Autodesk Fusion 360 part; units mm, degrees
(part 5 of 7)
  spline S1268 degree 3 poles (-26.8573, 27.0141) (-26.7843, 26.9991) (-26.7112, 26.9819) (-26.6403, 26.9626) knots 0 0 0 0 1 1 1 1
  spline S1269 degree 3 poles (-26.6403, 26.9626) (-26.7779, 27.1452) (-27.2419, 27.8115) (-27.359, 27.934) knots 0 0 0 0 1 1 1 1
  spline S1270 degree 3 poles (-27.359, 27.934) (-27.4804, 28.0619) (-27.4042, 28.1242) (-27.2967, 28.0114) knots 0 0 0 0 1 1 1 1
  spline S1271 degree 3 poles (-27.2967, 28.0114) (-27.2076, 27.9179) (-26.506, 27.1528) (-26.2332, 26.8132) knots 0 0 0 0 1 1 1 1
  spline S1272 degree 3 poles (-26.2332, 26.8132) (-26.159, 26.7767) (-26.086, 26.738) (-26.0172, 26.6939) knots 0 0 0 0 1 1 1 1
  line L670 (-26.0172, 26.6939) -> (-25.9807, 26.6692)
  spline S1273 degree 3 poles (-25.9807, 26.6692) (-26.0989, 26.8454) (-26.6231, 27.488) (-26.7305, 27.6535) knots 0 0 0 0 1 1 1 1
  spline S1274 degree 3 poles (-26.7305, 27.6535) (-26.8477, 27.833) (-26.7757, 27.8384) (-26.7037, 27.7492) knots 0 0 0 0 1 1 1 1
  spline S1275 degree 3 poles (-26.7037, 27.7492) (-26.6317, 27.661) (-25.8883, 26.8583) (-25.7755, 26.7412) knots 0 0 0 0 1 1 1 1
  spline S1276 degree 3 poles (-25.7755, 26.7412) (-25.7562, 26.7734) (-25.7368, 26.8089) (-25.7174, 26.8487) knots 0 0 0 0 1 1 1 1
  spline S1277 degree 3 poles (-25.7174, 26.8487) (-25.8603, 27.0163) (-26.5586, 27.8749) (-26.6532, 28.006) knots 0 0 0 0 1 1 1 1
  spline S1278 degree 3 poles (-26.6532, 28.006) (-26.7541, 28.1446) (-26.635, 28.1511) (-26.5802, 28.0672) knots 0 0 0 0 1 1 1 1
  spline S1279 degree 3 poles (-26.5802, 28.0672) (-26.5286, 27.9888) (-25.8356, 27.1882) (-25.6584, 26.9894) knots 0 0 0 0 1 1 1 1
  spline S1280 degree 3 poles (-25.6584, 26.9894) (-25.6391, 27.0335) (-25.6241, 27.0808) (-25.6058, 27.1324) knots 0 0 0 0 1 1 1 1
  spline S1281 degree 3 poles (-25.6058, 27.1324) (-25.6895, 27.2334) (-26.202, 27.8953) (-26.2793, 27.9888) knots 0 0 0 0 1 1 1 1
  spline S1282 degree 3 poles (-26.2793, 27.9888) (-26.3567, 28.0834) (-26.3061, 28.1285) (-26.2396, 28.0726) knots 0 0 0 0 1 1 1 1
  spline S1283 degree 3 poles (-26.2396, 28.0726) (-26.1729, 28.0167) (-25.6692, 27.3731) (-25.5853, 27.2667) knots 0 0 0 0 1 1 1 1
  line L671 (-25.5853, 27.2667) -> (-25.5714, 27.2506)
  spline S1284 degree 3 poles (-25.5714, 27.2506) (-25.5541, 27.3021) (-25.5413, 27.3591) (-25.5263, 27.4182) knots 0 0 0 0 1 1 1 1
  spline S1285 degree 3 poles (-25.5263, 27.4182) (-25.6252, 27.5686) (-25.8915, 27.9576) (-25.9592, 28.0715) knots 0 0 0 0 1 1 1 1
  spline S1286 degree 3 poles (-25.9592, 28.0715) (-26.0375, 28.2026) (-26.0258, 28.2188) (-25.9367, 28.1242) knots 0 0 0 0 1 1 1 1
  spline S1287 degree 3 poles (-25.9367, 28.1242) (-25.8614, 28.0436) (-25.5735, 27.7083) (-25.4832, 27.6019) knots 0 0 0 0 1 1 1 1
  spline S1288 degree 3 poles (-25.4832, 27.6019) (-25.4629, 27.6944) (-25.4447, 27.7943) (-25.4253, 27.9018) knots 0 0 0 0 1 1 1 1
  spline S1289 degree 3 poles (-25.4253, 27.9018) (-25.4457, 27.9308) (-25.4682, 27.9673) (-25.494, 28.0114) knots 0 0 0 0 1 1 1 1
  spline S1290 degree 3 poles (-25.494, 28.0114) (-25.536, 28.0866) (-25.466, 28.0425) (-25.4103, 27.9995) knots 0 0 0 0 1 1 1 1
  spline S1291 degree 3 poles (-25.4103, 27.9995) (-25.3791, 28.2059) (-25.348, 28.4412) (-25.3221, 28.7088) knots 0 0 0 0 1 1 1 1
  spline S1292 degree 3 poles (-25.3221, 28.7088) (-25.3469, 28.7442) (-25.3866, 28.7754) (-25.4543, 28.8678) knots 0 0 0 0 1 1 1 1
  spline S1293 degree 3 poles (-25.4543, 28.8678) (-25.5446, 28.9903) (-25.4198, 28.9409) (-25.3071, 28.8764) knots 0 0 0 0 1 1 1 1
  line L672 (-25.3071, 28.8764) -> (-25.2963, 28.9968)
  spline S1294 degree 3 poles (-25.2963, 28.9968) (-25.3264, 29.0387) (-25.3606, 29.0776) (-25.3984, 29.1128) knots 0 0 0 0 1 1 1 1
  spline S1295 degree 3 poles (-25.3984, 29.1128) (-25.4876, 29.1966) (-25.465, 29.2805) (-25.3813, 29.2203) knots 0 0 0 0 1 1 1 1
  spline S1296 degree 3 poles (-25.3813, 29.2203) (-25.3517, 29.1977) (-25.3188, 29.1803) (-25.2835, 29.1687) knots 0 0 0 0 1 1 1 1
  line L673 (-25.2835, 29.1687) -> (-25.2727, 29.3557)
  spline S1297 degree 3 poles (-25.2727, 29.3557) (-25.3447, 29.5029) (-25.4198, 29.6458) (-25.4865, 29.7845) knots 0 0 0 0 1 1 1 1
  spline S1298 degree 3 poles (-25.4865, 29.7845) (-25.5671, 29.9489) (-25.4779, 29.8984) (-25.422, 29.8253) knots 0 0 0 0 1 1 1 1
  spline S1299 degree 3 poles (-33.2215, 27.8308) (-33.1195, 27.6578) (-32.6929, 26.9884) (-32.4921, 26.7519) knots 0 0 0 0 1 1 1 1
  line L674 (-32.4921, 26.7519) -> (-32.3427, 26.7509)
  spline S1300 degree 3 poles (-32.3427, 26.7509) (-32.5276, 27.0034) (-33.0131, 27.6643) (-33.1313, 27.9566) knots 0 0 0 0 1 1 1 1
  spline S1301 degree 3 poles (-33.1313, 27.9566) (-33.1614, 27.9136) (-33.1904, 27.8717) (-33.2215, 27.8308) knots 0 0 0 0 1 1 1 1
  spline S1302 degree 3 poles (-33.445, 27.5719) (-33.3268, 27.4118) (-33.026, 26.9658) (-32.8595, 26.7562) knots 0 0 0 0 1 1 1 1
  line L675 (-32.8595, 26.7562) -> (-32.7328, 26.7541)
  spline S1303 degree 3 poles (-32.7328, 26.7541) (-32.8777, 26.955) (-33.2688, 27.5052) (-33.3569, 27.6654) knots 0 0 0 0 1 1 1 1
  spline S1304 degree 3 poles (-33.3569, 27.6654) (-33.3857, 27.6337) (-33.4151, 27.6025) (-33.445, 27.5719) knots 0 0 0 0 1 1 1 1
  spline S1305 degree 3 poles (-33.6491, 27.3892) (-33.5825, 27.2839) (-33.358, 26.9228) (-33.2247, 26.7627) knots 0 0 0 0 1 1 1 1
  spline S1306 degree 3 poles (-33.2247, 26.7627) (-33.1828, 26.7627) (-33.1409, 26.7627) (-33.099, 26.7605) knots 0 0 0 0 1 1 1 1
  spline S1307 degree 3 poles (-33.099, 26.7605) (-33.1904, 26.8852) (-33.4428, 27.2635) (-33.5707, 27.4536) knots 0 0 0 0 1 1 1 1
  spline S1308 degree 3 poles (-33.5707, 27.4536) (-33.5964, 27.4322) (-33.6222, 27.4096) (-33.6491, 27.3892) knots 0 0 0 0 1 1 1 1
  spline S1309 degree 3 poles (-29.8762, 30.2562) (-29.8095, 30.1111) (-29.7751, 29.9875) (-29.7247, 29.937) knots 0 0 0 0 1 1 1 1
  spline S1310 degree 3 poles (-29.7247, 29.937) (-29.6743, 29.8865) (-29.5571, 29.937) (-29.6237, 30.0542) knots 0 0 0 0 1 1 1 1
  spline S1311 degree 3 poles (-29.6237, 30.0542) (-29.6914, 30.1724) (-29.96, 30.441) (-29.8762, 30.2562) knots 0 0 0 0 1 1 1 1
  spline S1312 degree 3 poles (-29.9933, 29.8865) (-29.96, 29.8027) (-29.9094, 29.5341) (-29.9761, 29.6512) knots 0 0 0 0 1 1 1 1
  spline S1313 degree 3 poles (-29.9761, 29.6512) (-30.0426, 29.7694) (-30.178, 29.8693) (-30.0932, 29.9037) knots 0 0 0 0 1 1 1 1
  spline S1314 degree 2 poles (-30.0932, 29.9037) (-30.0105, 29.937) (-29.9933, 29.8865) knots 0 0 0 1 1 1
  spline S1315 degree 2 poles (-34.7277, 27.6374) (-34.6933, 27.4698) (-34.6267, 27.4698) knots 0 0 0 1 1 1
  spline S1316 degree 3 poles (-34.6267, 27.4698) (-34.5591, 27.4698) (-34.5311, 27.5471) (-34.7277, 27.6374) knots 0 0 0 0 1 1 1 1
  spline S1317 degree 2 poles (-34.442, 27.704) (-34.3915, 27.5536) (-34.3248, 27.6041) knots 0 0 0 1 1 1
  spline S1318 degree 3 poles (-34.3248, 27.6041) (-34.2572, 27.6535) (-34.3077, 27.6879) (-34.442, 27.704) knots 0 0 0 0 1 1 1 1
  spline S1319 degree 2 poles (-19.3845, 31.4974) (-19.5692, 31.6511) (-19.6703, 32.2023) knots 0 0 0 1 1 1
  spline S1320 degree 2 poles (-19.6703, 32.2023) (-19.7711, 32.759) (-19.9054, 33.162) knots 0 0 0 1 1 1
  spline S1321 degree 2 poles (-19.9054, 33.162) (-19.7368, 33.0427) (-19.5703, 32.4903) knots 0 0 0 1 1 1
  spline S1322 degree 3 poles (-19.5703, 32.4903) (-19.4017, 31.9348) (-19.2502, 31.4147) (-19.3845, 31.4974) knots 0 0 0 0 1 1 1 1
  spline S1323 degree 3 poles (-20.0837, 32.4441) (-20.1698, 32.9084) (-20.3159, 33.3381) (-20.3083, 33.3533) knots 0 0 0 0 1 1 1 1
  spline S1324 degree 3 poles (-20.3083, 33.3533) (-20.2997, 33.364) (-20.1515, 33.2436) (-20.0032, 32.7471) knots 0 0 0 0 1 1 1 1
  spline S1325 degree 3 poles (-20.0032, 32.7471) (-19.8572, 32.2561) (-19.7218, 31.7875) (-19.8389, 31.8488) knots 0 0 0 0 1 1 1 1
  spline S1326 degree 3 poles (-19.8389, 31.8488) (-19.8356, 31.8402) (-19.9957, 31.9659) (-20.0837, 32.4441) knots 0 0 0 0 1 1 1 1
  spline S1327 degree 3 poles (-20.4963, 32.6859) (-20.5683, 33.0599) (-20.7283, 33.5166) (-20.7111, 33.5424) knots 0 0 0 0 1 1 1 1
  spline S1328 degree 3 poles (-20.7111, 33.5424) (-20.694, 33.5692) (-20.5641, 33.4457) (-20.4384, 33.005) knots 0 0 0 0 1 1 1 1
  spline S1329 degree 3 poles (-20.4384, 33.005) (-20.3127, 32.5752) (-20.1923, 32.1593) (-20.29, 32.1991) knots 0 0 0 0 1 1 1 1
  spline S1330 degree 3 poles (-20.29, 32.1991) (-20.2869, 32.1841) (-20.4223, 32.2808) (-20.4963, 32.6859) knots 0 0 0 0 1 1 1 1
  spline S1331 degree 3 poles (-20.9099, 32.9267) (-20.9669, 33.2124) (-21.1388, 33.6971) (-21.1131, 33.7325) knots 0 0 0 0 1 1 1 1
  spline S1332 degree 3 poles (-21.1131, 33.7325) (-21.0882, 33.7702) (-20.9766, 33.6465) (-20.8714, 33.2641) knots 0 0 0 0 1 1 1 1
  spline S1333 degree 3 poles (-20.8714, 33.2641) (-20.7649, 32.8965) (-20.6651, 32.5311) (-20.7413, 32.5505) knots 0 0 0 0 1 1 1 1
  spline S1334 degree 3 poles (-20.7413, 32.5505) (-20.738, 32.5236) (-20.8487, 32.5956) (-20.9099, 32.9267) knots 0 0 0 0 1 1 1 1
  spline S1335 degree 3 poles (-21.3236, 33.1706) (-21.3654, 33.3618) (-21.5503, 33.8734) (-21.5169, 33.926) knots 0 0 0 0 1 1 1 1
  spline S1336 degree 3 poles (-21.5169, 33.926) (-21.4836, 33.9764) (-21.3902, 33.8486) (-21.3075, 33.523) knots 0 0 0 0 1 1 1 1
  spline S1337 degree 3 poles (-21.3075, 33.523) (-21.2236, 33.2168) (-21.1388, 32.9062) (-21.1957, 32.8998) knots 0 0 0 0 1 1 1 1
  spline S1338 degree 3 poles (-21.1957, 32.8998) (-21.1882, 32.8664) (-21.2752, 32.9104) (-21.3236, 33.1706) knots 0 0 0 0 1 1 1 1
  spline S1339 degree 3 poles (-21.7372, 33.4101) (-21.7641, 33.5133) (-21.9617, 34.0528) (-21.9197, 34.1173) knots 0 0 0 0 1 1 1 1
  spline S1340 degree 3 poles (-21.9197, 34.1173) (-21.8779, 34.1785) (-21.8048, 34.0506) (-21.7414, 33.7799) knots 0 0 0 0 1 1 1 1
  spline S1341 degree 3 poles (-21.7414, 33.7799) (-21.678, 33.538) (-21.6093, 33.2758) (-21.648, 33.2511) knots 0 0 0 0 1 1 1 1
  spline S1342 degree 3 poles (-21.648, 33.2511) (-21.6395, 33.2082) (-21.7018, 33.2254) (-21.7372, 33.4101) knots 0 0 0 0 1 1 1 1
  spline S1343 degree 3 poles (-22.1497, 33.6509) (-22.1636, 33.6659) (-22.3732, 34.23) (-22.3226, 34.3053) knots 0 0 0 0 1 1 1 1
  spline S1344 degree 3 poles (-22.3226, 34.3053) (-22.2722, 34.3827) (-22.2174, 34.2505) (-22.1755, 34.0367) knots 0 0 0 0 1 1 1 1
  spline S1345 degree 3 poles (-22.1755, 34.0367) (-22.1337, 33.8561) (-22.0809, 33.6487) (-22.1002, 33.6004) knots 0 0 0 0 1 1 1 1
  spline S1346 degree 3 poles (-22.1002, 33.6004) (-22.0906, 33.5477) (-22.1271, 33.5402) (-22.1497, 33.6509) knots 0 0 0 0 1 1 1 1
  spline S1347 degree 3 poles (-22.5634, 33.8948) (-22.5612, 33.8153) (-22.7836, 34.4096) (-22.7245, 34.4977) knots 0 0 0 0 1 1 1 1
  spline S1348 degree 3 poles (-22.7245, 34.4977) (-22.6654, 34.5857) (-22.6299, 34.4536) (-22.6095, 34.2978) knots 0 0 0 0 1 1 1 1
  spline S1349 degree 3 poles (-22.6095, 34.2978) (-22.5881, 34.1763) (-22.5515, 34.0227) (-22.5526, 33.9518) knots 0 0 0 0 1 1 1 1
  spline S1350 degree 3 poles (-22.5526, 33.9518) (-22.5418, 33.8926) (-22.5537, 33.8551) (-22.5634, 33.8948) knots 0 0 0 0 1 1 1 1
  spline S1351 degree 3 poles (-22.9769, 34.1334) (-22.9586, 33.9679) (-23.195, 34.5868) (-23.1283, 34.69) knots 0 0 0 0 1 1 1 1
  spline S1352 degree 3 poles (-23.1283, 34.69) (-23.0618, 34.7889) (-23.0446, 34.6546) (-23.0446, 34.5558) knots 0 0 0 0 1 1 1 1
  spline S1353 degree 3 poles (-23.0446, 34.5558) (-23.0446, 34.4525) (-22.9855, 34.2172) (-22.9769, 34.1334) knots 0 0 0 0 1 1 1 1
  spline S1354 degree 3 poles (-23.3271, 34.2934) (-23.3121, 34.1484) (-23.5259, 34.7363) (-23.4786, 34.8351) knots 0 0 0 0 1 1 1 1
  spline S1355 degree 3 poles (-23.4786, 34.8351) (-23.426, 34.9296) (-23.3969, 34.8104) (-23.3872, 34.7072) knots 0 0 0 0 1 1 1 1
  spline S1356 degree 3 poles (-23.3872, 34.7072) (-23.3808, 34.6084) (-23.3249, 34.3881) (-23.3271, 34.2934) knots 0 0 0 0 1 1 1 1
  spline S1357 degree 3 poles (-23.6774, 34.4504) (-23.6645, 34.3332) (-23.8557, 34.8802) (-23.8277, 34.9813) knots 0 0 0 0 1 1 1 1
  spline S1358 degree 3 poles (-23.8277, 34.9813) (-23.7912, 35.0693) (-23.7493, 34.9641) (-23.73, 34.8598) knots 0 0 0 0 1 1 1 1
  spline S1359 degree 3 poles (-23.73, 34.8598) (-23.7172, 34.7609) (-23.6677, 34.56) (-23.6774, 34.4504) knots 0 0 0 0 1 1 1 1
  spline S1360 degree 3 poles (-24.0265, 34.6106) (-24.0179, 34.5138) (-24.1876, 35.0286) (-24.1791, 35.1285) knots 0 0 0 0 1 1 1 1
  spline S1361 degree 3 poles (-24.1791, 35.1285) (-24.1575, 35.2102) (-24.1029, 35.1199) (-24.0738, 35.0112) knots 0 0 0 0 1 1 1 1
  spline S1362 degree 3 poles (-24.0738, 35.0112) (-24.0534, 34.9168) (-24.0082, 34.7297) (-24.0265, 34.6106) knots 0 0 0 0 1 1 1 1
  spline S1363 degree 3 poles (-24.3778, 34.7673) (-24.3703, 34.6965) (-24.5185, 35.1726) (-24.5282, 35.2756) knots 0 0 0 0 1 1 1 1
  spline S1364 degree 3 poles (-24.5282, 35.2756) (-24.5229, 35.3509) (-24.4551, 35.2756) (-24.4166, 35.1629) knots 0 0 0 0 1 1 1 1
  spline S1365 degree 3 poles (-24.4166, 35.1629) (-24.3897, 35.0693) (-24.3488, 34.8974) (-24.3778, 34.7673) knots 0 0 0 0 1 1 1 1
  spline S1366 degree 3 poles (-24.727, 34.9276) (-24.7226, 34.8791) (-24.8494, 35.3198) (-24.8785, 35.4207) knots 0 0 0 0 1 1 1 1
  spline S1367 degree 3 poles (-24.8785, 35.4207) (-24.887, 35.4917) (-24.8076, 35.4293) (-24.7592, 35.3132) knots 0 0 0 0 1 1 1 1
  spline S1368 degree 3 poles (-24.7592, 35.3132) (-24.7115, 35.1905) (-24.7003, 35.0565) (-24.727, 34.9276) knots 0 0 0 0 1 1 1 1
  spline S1369 degree 3 poles (-25.0772, 35.0843) (-25.075, 35.0618) (-25.1803, 35.4658) (-25.2287, 35.5668) knots 0 0 0 0 1 1 1 1
  spline S1370 degree 3 poles (-25.2287, 35.5668) (-25.2534, 35.6324) (-25.1598, 35.584) (-25.1019, 35.4638) knots 0 0 0 0 1 1 1 1
  spline S1371 degree 3 poles (-25.1019, 35.4638) (-25.0487, 35.3443) (-25.0399, 35.2097) (-25.0772, 35.0843) knots 0 0 0 0 1 1 1 1
  spline S1372 degree 2 poles (-25.4275, 35.2423) (-25.5112, 35.612) (-25.5789, 35.713) knots 0 0 0 1 1 1
  spline S1373 degree 3 poles (-25.5789, 35.713) (-25.6455, 35.8151) (-25.2932, 35.6454) (-25.4275, 35.2423) knots 0 0 0 0 1 1 1 1
  spline S1374 degree 2 poles (-19.1835, 28.611) (-19.3683, 29.0473) (-19.4017, 29.4503) knots 0 0 0 1 1 1
  spline S1375 degree 3 poles (-19.4017, 29.4503) (-19.4349, 29.8533) (-19.5864, 30.8773) (-19.7874, 31.0955) knots 0 0 0 0 1 1 1 1
  spline S1376 degree 3 poles (-19.7874, 31.0955) (-19.9882, 31.3136) (-19.6863, 31.2126) (-19.6014, 31.0289) knots 0 0 0 0 1 1 1 1
  spline S1377 degree 3 poles (-19.6014, 31.0289) (-19.5188, 30.8451) (-19.2329, 29.8199) (-19.2329, 29.4514) knots 0 0 0 0 1 1 1 1
  spline S1378 degree 2 poles (-19.2329, 29.4514) (-19.234, 29.0817) (-19.1835, 28.611) knots 0 0 0 1 1 1
  spline S1379 degree 2 poles (-19.536, 28.7454) (-19.8711, 29.0473) (-19.9098, 29.6684) knots 0 0 0 1 1 1
  spline S1380 degree 3 poles (-19.9098, 29.6684) (-19.9334, 30.0725) (-20.0569, 31.0955) (-20.2578, 31.3136) knots 0 0 0 0 1 1 1 1
  spline S1381 degree 3 poles (-20.2578, 31.3136) (-20.4597, 31.5318) (-20.1944, 31.4308) (-20.1106, 31.247) knots 0 0 0 0 1 1 1 1
  spline S1382 degree 3 poles (-20.1106, 31.247) (-20.0269, 31.0622) (-19.7411, 30.0381) (-19.7411, 29.6684) knots 0 0 0 0 1 1 1 1
  spline S1383 degree 2 poles (-19.7411, 29.6684) (-19.7411, 29.2988) (-19.536, 28.7454) knots 0 0 0 1 1 1
  spline S1384 degree 2 poles (-19.9957, 29.1537) (-20.3148, 29.4589) (-20.3545, 30.0413) knots 0 0 0 1 1 1
  spline S1385 degree 3 poles (-20.3545, 30.0413) (-20.3814, 30.426) (-20.4877, 31.3878) (-20.6823, 31.5984) knots 0 0 0 0 1 1 1 1
  spline S1386 degree 3 poles (-20.6823, 31.5984) (-20.8648, 31.7961) (-20.607, 31.665) (-20.5286, 31.4813) knots 0 0 0 0 1 1 1 1
  spline S1387 degree 3 poles (-20.5286, 31.4813) (-20.4512, 31.3018) (-20.1891, 30.3583) (-20.187, 30.0102) knots 0 0 0 0 1 1 1 1
  spline S1388 degree 3 poles (-20.187, 30.0102) (-20.1837, 29.6674) (-19.9968, 29.158) (-19.9957, 29.1537) knots 0 0 0 0 1 1 1 1
  spline S1389 degree 2 poles (-20.5317, 29.7522) (-20.8368, 30.0574) (-20.8778, 30.6023) knots 0 0 0 1 1 1
  spline S1390 degree 3 poles (-20.8778, 30.6023) (-20.9068, 30.9698) (-20.996, 31.8692) (-21.184, 32.0701) knots 0 0 0 0 1 1 1 1
  spline S1391 degree 3 poles (-21.184, 32.0701) (-21.3482, 32.2485) (-21.0957, 32.0873) (-21.0238, 31.9025) knots 0 0 0 0 1 1 1 1
  spline S1392 degree 3 poles (-21.0238, 31.9025) (-20.9529, 31.7306) (-20.7155, 30.8655) (-20.7102, 30.5399) knots 0 0 0 0 1 1 1 1
  spline S1393 degree 3 poles (-20.7102, 30.5399) (-20.7069, 30.2261) (-20.535, 29.7598) (-20.5317, 29.7522) knots 0 0 0 0 1 1 1 1
  spline S1394 degree 3 poles (-21.923, 31.6113) (-21.8952, 31.3276) (-21.785, 31.0583) (-21.606, 30.8365) knots 0 0 0 0 1 1 1 1
  spline S1395 degree 3 poles (-21.606, 30.8365) (-21.6137, 30.8526) (-21.75, 31.2277) (-21.7566, 31.4877) knots 0 0 0 0 1 1 1 1
  spline S1396 degree 3 poles (-21.7566, 31.4877) (-21.7683, 31.7693) (-21.9585, 32.4742) (-22.0144, 32.6354) knots 0 0 0 0 1 1 1 1
  spline S1397 degree 3 poles (-22.0144, 32.6354) (-22.0756, 32.8202) (-22.3151, 33.0427) (-22.1874, 32.904) knots 0 0 0 0 1 1 1 1
  spline S1398 degree 3 poles (-22.1874, 32.904) (-22.0166, 32.7149) (-21.9574, 31.9423) (-21.923, 31.6113) knots 0 0 0 0 1 1 1 1
  spline S1399 degree 3 poles (-22.0595, 31.1804) (-22.067, 31.2019) (-22.1883, 31.5318) (-22.196, 31.766) knots 0 0 0 0 1 1 1 1
  spline S1400 degree 3 poles (-22.196, 31.766) (-22.2099, 32.0239) (-22.3754, 32.6515) (-22.4258, 32.8052) knots 0 0 0 0 1 1 1 1
  spline S1401 degree 3 poles (-22.4258, 32.8052) (-22.4572, 32.8939) (-22.5022, 32.9772) (-22.559, 33.0524) knots 0 0 0 0 1 1 1 1
  spline S1402 degree 3 poles (-22.559, 33.0524) (-22.4344, 32.8052) (-22.3957, 32.2002) (-22.3624, 31.9208) knots 0 0 0 0 1 1 1 1
  spline S1403 degree 3 poles (-22.3624, 31.9208) (-22.3296, 31.6513) (-22.225, 31.3956) (-22.0595, 31.1804) knots 0 0 0 0 1 1 1 1
  spline S1404 degree 3 poles (-22.5172, 31.6532) (-22.5278, 31.6758) (-22.631, 31.9638) (-22.6407, 32.1712) knots 0 0 0 0 1 1 1 1
  spline S1405 degree 3 poles (-22.6407, 32.1712) (-22.6568, 32.4065) (-22.7985, 32.9546) (-22.8426, 33.1006) knots 0 0 0 0 1 1 1 1
  spline S1406 degree 3 poles (-22.8426, 33.1006) (-22.863, 33.1781) (-22.9146, 33.2727) (-22.9597, 33.35) knots 0 0 0 0 1 1 1 1
  spline S1407 degree 3 poles (-22.9597, 33.35) (-22.863, 33.0942) (-22.8384, 32.601) (-22.8051, 32.3571) knots 0 0 0 0 1 1 1 1
  spline S1408 degree 3 poles (-22.8051, 32.3571) (-22.7687, 32.1023) (-22.6697, 31.8604) (-22.5172, 31.6532) knots 0 0 0 0 1 1 1 1
  spline S1409 degree 3 poles (-22.9469, 31.9444) (-22.9575, 31.9713) (-23.0446, 32.2131) (-23.0554, 32.3936) knots 0 0 0 0 1 1 1 1
  spline S1410 degree 3 poles (-23.0554, 32.3936) (-23.0746, 32.6074) (-23.1939, 33.0759) (-23.2294, 33.219) knots 0 0 0 0 1 1 1 1
  spline S1411 degree 3 poles (-23.2294, 33.219) (-23.2487, 33.2963) (-23.2981, 33.3995) (-23.3454, 33.4854) knots 0 0 0 0 1 1 1 1
  spline S1412 degree 3 poles (-23.3454, 33.4854) (-23.2681, 33.2393) (-23.2529, 32.8288) (-23.2208, 32.6128) knots 0 0 0 0 1 1 1 1
  spline S1413 degree 2 poles (-23.2208, 32.6128) (-23.1746, 32.2571) (-22.9469, 31.9444) knots 0 0 0 1 1 1
  spline S1414 degree 3 poles (-23.4893, 32.5011) (-23.5034, 32.5322) (-23.5732, 32.7299) (-23.586, 32.8825) knots 0 0 0 0 1 1 1 1
  spline S1415 degree 3 poles (-23.586, 32.8825) (-23.6076, 33.0737) (-23.702, 33.4618) (-23.7333, 33.5961) knots 0 0 0 0 1 1 1 1
  spline S1416 degree 3 poles (-23.7333, 33.5961) (-23.7493, 33.6799) (-23.802, 33.7992) (-23.8515, 33.8959) knots 0 0 0 0 1 1 1 1
  spline S1417 degree 3 poles (-23.8515, 33.8959) (-23.7892, 33.6691) (-23.7837, 33.3231) (-23.7504, 33.1296) knots 0 0 0 0 1 1 1 1
  spline S1418 degree 2 poles (-23.7504, 33.1296) (-23.7042, 32.8159) (-23.4893, 32.5011) knots 0 0 0 1 1 1
  spline S1419 degree 3 poles (-23.9384, 32.8536) (-23.9545, 32.8868) (-24.006, 33.0427) (-24.0201, 33.1684) knots 0 0 0 0 1 1 1 1
  spline S1420 degree 3 poles (-24.0201, 33.1684) (-24.0437, 33.3361) (-24.1146, 33.6445) (-24.1383, 33.7744) knots 0 0 0 0 1 1 1 1
  spline S1421 degree 3 poles (-24.1383, 33.7744) (-24.1533, 33.8668) (-24.2145, 34.0077) (-24.2671, 34.1204) knots 0 0 0 0 1 1 1 1
  spline S1422 degree 3 poles (-24.2671, 34.1204) (-24.2167, 33.9174) (-24.2167, 33.6207) (-24.1844, 33.4466) knots 0 0 0 0 1 1 1 1
  spline S1423 degree 2 poles (-24.1844, 33.4466) (-24.1372, 33.1706) (-23.9384, 32.8536) knots 0 0 0 1 1 1
  spline S1424 degree 3 poles (-24.2693, 33.1684) (-24.2865, 33.206) (-24.3219, 33.3156) (-24.3369, 33.4145) knots 0 0 0 0 1 1 1 1
  spline S1425 degree 3 poles (-24.3369, 33.4145) (-24.3628, 33.5639) (-24.41, 33.7927) (-24.4283, 33.9141) knots 0 0 0 0 1 1 1 1
  spline S1426 degree 3 poles (-24.4283, 33.9141) (-24.4412, 34.0194) (-24.511, 34.1935) (-24.568, 34.3214) knots 0 0 0 0 1 1 1 1
  spline S1427 degree 3 poles (-24.568, 34.3214) (-24.5271, 34.1387) (-24.5368, 33.8873) (-24.5014, 33.725) knots 0 0 0 0 1 1 1 1
  spline S1428 degree 2 poles (-24.5014, 33.725) (-24.4529, 33.4854) (-24.2693, 33.1684) knots 0 0 0 1 1 1
  spline S1429 degree 3 poles (-24.8613, 34.2934) (-24.8269, 34.1345) (-24.843, 33.913) (-24.8065, 33.7647) knots 0 0 0 0 1 1 1 1
  spline S1430 degree 3 poles (-24.8065, 33.7647) (-24.7492, 33.5853) (-24.6762, 33.4113) (-24.5883, 33.2447) knots 0 0 0 0 1 1 1 1
  spline S1431 degree 3 poles (-24.5883, 33.2447) (-24.6389, 33.3618) (-24.6894, 33.6304) (-24.7043, 33.8153) knots 0 0 0 0 1 1 1 1
  spline S1432 degree 3 poles (-24.7043, 33.8153) (-24.7162, 33.9324) (-24.799, 34.1484) (-24.8613, 34.2934) knots 0 0 0 0 1 1 1 1
  spline S1433 degree 3 poles (-25.2512, 38.8648) (-25.2813, 38.5102) (-25.0889, 37.8149) (-25.0418, 37.7731) knots 0 0 0 0 1 1 1 1
  spline S1434 degree 3 poles (-25.0418, 37.7731) (-24.9289, 37.788) (-24.9998, 38.0943) (-25.1052, 38.9776) knots 0 0 0 0 1 1 1 1
  spline S1435 degree 3 poles (-25.1052, 38.9776) (-25.1986, 39.7685) (-25.4521, 39.7245) (-25.494, 39.7223) knots 0 0 0 0 1 1 1 1
  spline S1436 degree 3 poles (-25.494, 39.7223) (-25.4532, 39.6826) (-25.2232, 39.1937) (-25.2512, 38.8648) knots 0 0 0 0 1 1 1 1
  spline S1437 degree 3 poles (-24.8741, 38.81) (-24.902, 38.4823) (-24.7506, 37.8697) (-24.6561, 37.7859) knots 0 0 0 0 1 1 1 1
  spline S1438 degree 3 poles (-24.6561, 37.7859) (-24.5658, 37.7944) (-24.6389, 38.074) (-24.7323, 38.8164) knots 0 0 0 0 1 1 1 1
  spline S1439 degree 3 poles (-24.7323, 38.8164) (-24.799, 39.3645) (-24.9557, 39.4398) (-25.0213, 39.457) knots 0 0 0 0 1 1 1 1
  spline S1440 degree 3 poles (-25.0213, 39.457) (-24.9153, 39.2583) (-24.8644, 39.0349) (-24.8741, 38.81) knots 0 0 0 0 1 1 1 1
  spline S1441 degree 3 poles (-24.4626, 38.7509) (-24.4875, 38.4596) (-24.3789, 37.9223) (-24.2361, 37.7935) knots 0 0 0 0 1 1 1 1
  spline S1442 degree 3 poles (-24.2361, 37.7935) (-24.1683, 37.8021) (-24.2457, 38.0535) (-24.3263, 38.6542) knots 0 0 0 0 1 1 1 1
  spline S1443 degree 3 poles (-24.3263, 38.6542) (-24.3682, 38.9798) (-24.4465, 39.1013) (-24.5035, 39.1561) knots 0 0 0 0 1 1 1 1
  spline S1444 degree 3 poles (-24.5035, 39.1561) (-24.4745, 39.0636) (-24.4487, 38.9089) (-24.4626, 38.7509) knots 0 0 0 0 1 1 1 1
  spline S1445 degree 3 poles (-24.0512, 38.6961) (-24.0738, 38.4317) (-24.006, 37.974) (-23.816, 37.8063) knots 0 0 0 0 1 1 1 1
  spline S1446 degree 3 poles (-23.816, 37.8063) (-23.7698, 37.8107) (-23.8504, 38.033) (-23.9202, 38.4951) knots 0 0 0 0 1 1 1 1
  spline S1447 degree 3 poles (-23.9202, 38.4951) (-23.9503, 38.7218) (-24.004, 38.8228) (-24.0437, 38.8766) knots 0 0 0 0 1 1 1 1
  spline S1448 degree 3 poles (-24.0437, 38.8766) (-24.0434, 38.8164) (-24.0459, 38.7562) (-24.0512, 38.6961) knots 0 0 0 0 1 1 1 1
  spline S1449 degree 3 poles (-23.3626, 37.8171) (-23.6021, 38.0266) (-23.6258, 38.4092) (-23.6076, 38.6423) knots 0 0 0 0 1 1 1 1
  spline S1450 degree 3 poles (-23.6076, 38.6423) (-23.586, 38.8734) (-23.5345, 38.9025) (-23.5763, 38.7057) knots 0 0 0 0 1 1 1 1
  spline S1451 degree 3 poles (-23.5763, 38.7057) (-23.5915, 38.6392) (-23.5215, 38.5844) (-23.4819, 38.3339) knots 0 0 0 0 1 1 1 1
  spline S1452 degree 3 poles (-23.4819, 38.3339) (-23.4238, 38.0126) (-23.3401, 37.8193) (-23.3626, 37.8171) knots 0 0 0 0 1 1 1 1
  spline S1453 degree 2 poles (-22.9769, 31.4748) (-23.5474, 31.8714) (-23.9503, 32.2012) knots 0 0 0 1 1 1
  spline S1454 degree 3 poles (-23.9503, 32.2012) (-24.3532, 32.5322) (-23.2789, 31.8402) (-22.9769, 31.4748) knots 0 0 0 0 1 1 1 1
  spline S1455 degree 2 poles (-22.4397, 24.8908) (-23.0103, 25.2884) (-23.4131, 25.6183) knots 0 0 0 1 1 1
  spline S1456 degree 3 poles (-23.4131, 25.6183) (-23.816, 25.9493) (-22.7417, 25.2572) (-22.4397, 24.8908) knots 0 0 0 0 1 1 1 1
  spline S1457 degree 2 poles (-22.4903, 24.6963) (-23.0607, 25.095) (-23.4636, 25.4259) knots 0 0 0 1 1 1
  spline S1458 degree 3 poles (-23.4636, 25.4259) (-23.8665, 25.7558) (-22.7921, 25.0638) (-22.4903, 24.6963) knots 0 0 0 0 1 1 1 1
  spline S1459 degree 2 poles (-22.3688, 24.2363) (-22.9394, 24.634) (-23.3423, 24.9649) knots 0 0 0 1 1 1
  spline S1460 degree 3 poles (-23.3423, 24.9649) (-23.7451, 25.2959) (-22.6708, 24.6039) (-22.3688, 24.2363) knots 0 0 0 0 1 1 1 1
  spline S1461 degree 2 poles (-22.6621, 24.173) (-23.2316, 24.5706) (-23.6344, 24.9015) knots 0 0 0 1 1 1
  spline S1462 degree 3 poles (-23.6344, 24.9015) (-24.0373, 25.2314) (-22.963, 24.5405) (-22.6621, 24.173) knots 0 0 0 0 1 1 1 1
  spline S1463 degree 2 poles (-23.3658, 24.3041) (-23.9373, 24.7016) (-24.3402, 25.0326) knots 0 0 0 1 1 1
  spline S1464 degree 3 poles (-24.3402, 25.0326) (-24.7431, 25.3636) (-23.6699, 24.6716) (-23.3658, 24.3041) knots 0 0 0 0 1 1 1 1
  spline S1465 degree 2 poles (-23.4894, 25.2927) (-23.8825, 25.5828) (-24.1608, 25.8246) knots 0 0 0 1 1 1
  spline S1466 degree 3 poles (-24.1608, 25.8246) (-24.4369, 26.0664) (-23.6967, 25.5624) (-23.4894, 25.2927) knots 0 0 0 0 1 1 1 1
  spline S1467 degree 2 poles (-23.7472, 25.8665) (-24.1403, 26.1567) (-24.4186, 26.3984) knots 0 0 0 1 1 1
  spline S1468 degree 3 poles (-24.4186, 26.3984) (-24.6969, 26.6402) (-23.9556, 26.1352) (-23.7472, 25.8665) knots 0 0 0 0 1 1 1 1
  spline S1469 degree 2 poles (-22.963, 31.1782) (-23.9836, 31.9219) (-24.3864, 32.2517) knots 0 0 0 1 1 1
  spline S1470 degree 3 poles (-24.3864, 32.2517) (-24.7904, 32.5827) (-23.267, 31.5458) (-22.963, 31.1782) knots 0 0 0 0 1 1 1 1
  spline S1471 degree 2 poles (-22.8674, 30.7925) (-23.888, 31.5339) (-24.2909, 31.866) knots 0 0 0 1 1 1
  spline S1472 degree 3 poles (-24.2909, 31.866) (-24.6937, 32.198) (-23.1703, 31.1589) (-22.8674, 30.7925) knots 0 0 0 0 1 1 1 1
  spline S1473 degree 2 poles (-22.9876, 26.8326) (-24.0071, 27.5762) (-24.41, 27.9061) knots 0 0 0 1 1 1
  spline S1474 degree 3 poles (-24.41, 27.9061) (-24.8129, 28.2381) (-23.2895, 27.2001) (-22.9876, 26.8326) knots 0 0 0 0 1 1 1 1
  spline S1475 degree 2 poles (-23.138, 26.6219) (-24.1586, 27.3645) (-24.5615, 27.6966) knots 0 0 0 1 1 1
  spline S1476 degree 3 poles (-24.5615, 27.6966) (-24.9643, 28.0264) (-23.4409, 26.9895) (-23.138, 26.6219) knots 0 0 0 0 1 1 1 1
  spline S1477 degree 2 poles (-22.2046, 29.6749) (-23.9437, 30.9719) (-24.3466, 31.3029) knots 0 0 0 1 1 1
  spline S1478 degree 3 poles (-24.3466, 31.3029) (-24.7495, 31.6339) (-22.5075, 30.0424) (-22.2046, 29.6749) knots 0 0 0 0 1 1 1 1
  spline S1479 degree 2 poles (-22.0305, 25.2873) (-23.7698, 26.5843) (-24.1727, 26.9153) knots 0 0 0 1 1 1
  spline S1480 degree 3 poles (-24.1727, 26.9153) (-24.5755, 27.2452) (-22.3323, 25.6548) (-22.0305, 25.2873) knots 0 0 0 0 1 1 1 1
  spline S1481 degree 2 poles (-22.1229, 25.0272) (-23.8621, 26.3243) (-24.2649, 26.6553) knots 0 0 0 1 1 1
  spline S1482 degree 3 poles (-24.2649, 26.6553) (-24.6678, 26.9862) (-22.4247, 25.3948) (-22.1229, 25.0272) knots 0 0 0 0 1 1 1 1
  spline S1483 degree 2 poles (-22.1088, 29.3192) (-23.8471, 30.6162) (-24.25, 30.9472) knots 0 0 0 1 1 1
  spline S1484 degree 3 poles (-24.25, 30.9472) (-24.6528, 31.2782) (-22.4108, 29.6856) (-22.1088, 29.3192) knots 0 0 0 0 1 1 1 1
  spline S1485 degree 2 poles (-22.0917, 28.9635) (-23.831, 30.2616) (-24.2339, 30.5915) knots 0 0 0 1 1 1
  spline S1486 degree 3 poles (-24.2339, 30.5915) (-24.6367, 30.9236) (-22.3935, 29.331) (-22.0917, 28.9635) knots 0 0 0 0 1 1 1 1
  spline S1487 degree 2 poles (-22.024, 28.6508) (-23.7623, 29.9478) (-24.1652, 30.2788) knots 0 0 0 1 1 1
  spline S1488 degree 3 poles (-24.1652, 30.2788) (-24.569, 30.6098) (-22.327, 29.0172) (-22.024, 28.6508) knots 0 0 0 0 1 1 1 1
  spline S1489 degree 2 poles (-22.1271, 28.4133) (-23.8665, 29.7103) (-24.2693, 30.0413) knots 0 0 0 1 1 1
  spline S1490 degree 3 poles (-24.2693, 30.0413) (-24.6722, 30.3723) (-22.4291, 28.7808) (-22.1271, 28.4133) knots 0 0 0 0 1 1 1 1
  spline S1491 degree 2 poles (-22.1088, 27.516) (-23.8471, 28.8141) (-24.25, 29.144) knots 0 0 0 1 1 1
  spline S1492 degree 3 poles (-24.25, 29.144) (-24.6528, 29.475) (-22.4108, 27.8835) (-22.1088, 27.516) knots 0 0 0 0 1 1 1 1
  spline S1493 degree 2 poles (-22.0745, 27.1915) (-23.8138, 28.4885) (-24.2167, 28.8206) knots 0 0 0 1 1 1
  spline S1494 degree 3 poles (-24.2167, 28.8206) (-24.6196, 29.1505) (-22.3763, 27.559) (-22.0745, 27.1915) knots 0 0 0 0 1 1 1 1
  spline S1495 degree 2 poles (-21.9574, 26.8025) (-23.6967, 28.1006) (-24.0996, 28.4316) knots 0 0 0 1 1 1
  spline S1496 degree 3 poles (-24.0996, 28.4316) (-24.5024, 28.7625) (-22.2592, 27.1711) (-21.9574, 26.8025) knots 0 0 0 0 1 1 1 1
  spline S1497 degree 2 poles (-22.226, 26.7455) (-23.9653, 28.0436) (-24.3682, 28.3746) knots 0 0 0 1 1 1
  spline S1498 degree 3 poles (-24.3682, 28.3746) (-24.771, 28.7045) (-22.5278, 27.1141) (-22.226, 26.7455) knots 0 0 0 0 1 1 1 1
  spline S1499 degree 2 poles (-21.9906, 26.2716) (-23.73, 27.5687) (-24.1328, 27.8996) knots 0 0 0 1 1 1
  spline S1500 degree 3 poles (-24.1328, 27.8996) (-24.5357, 28.2306) (-22.2926, 26.6391) (-21.9906, 26.2716) knots 0 0 0 0 1 1 1 1
  spline S1501 degree 2 poles (-21.9928, 27.9899) (-23.2025, 28.8861) (-23.8986, 29.4589) knots 0 0 0 1 1 1
  spline S1502 degree 3 poles (-23.8986, 29.4589) (-24.3026, 29.7888) (-22.2948, 28.3574) (-21.9928, 27.9899) knots 0 0 0 0 1 1 1 1
  spline S1503 degree 2 poles (-22.24, 27.8663) (-23.4497, 28.7626) (-24.148, 29.3353) knots 0 0 0 1 1 1
  spline S1504 degree 3 poles (-24.148, 29.3353) (-24.5509, 29.6663) (-22.5429, 28.2338) (-22.24, 27.8663) knots 0 0 0 0 1 1 1 1
  spline S1505 degree 2 poles (-23.1283, 30.6796) (-23.7826, 31.1363) (-24.1855, 31.4684) knots 0 0 0 1 1 1
  spline S1506 degree 3 poles (-24.1855, 31.4684) (-24.5883, 31.7983) (-23.4303, 31.0482) (-23.1283, 30.6796) knots 0 0 0 0 1 1 1 1
  spline S1507 degree 2 poles (-22.1883, 29.8275) (-22.4183, 29.9682) (-22.8212, 30.2992) knots 0 0 0 1 1 1
  spline S1508 degree 3 poles (-22.8212, 30.2992) (-23.2241, 30.6291) (-22.4903, 30.195) (-22.1883, 29.8275) knots 0 0 0 0 1 1 1 1
  spline S1509 degree 2 poles (-22.024, 28.6465) (-23.6236, 29.8286) (-24.1652, 30.2735) knots 0 0 0 1 1 1
  line L676 (-24.1652, 30.2735) -> (-22.024, 28.6465)
  spline S1510 degree 2 poles (-20.7466, 34.7889) (-20.7005, 34.8985) (-20.7166, 35.5992) knots 0 0 0 1 1 1
  spline S1511 degree 3 poles (-20.7166, 35.5992) (-20.7182, 35.7216) (-20.7294, 35.8438) (-20.7499, 35.9645) knots 0 0 0 0 1 1 1 1
  spline S1512 degree 3 poles (-20.7499, 35.9645) (-20.8144, 36.0634) (-20.8788, 36.158) (-20.9465, 36.2547) knots 0 0 0 0 1 1 1 1
  spline S1513 degree 3 poles (-20.9465, 36.2547) (-20.9143, 35.9505) (-20.8842, 35.4992) (-20.8842, 35.2747) knots 0 0 0 0 1 1 1 1
  spline S1514 degree 3 poles (-20.8842, 35.2747) (-20.887, 35.1028) (-20.8392, 34.9338) (-20.7466, 34.7889) knots 0 0 0 0 1 1 1 1
  spline S1515 degree 2 poles (-20.362, 34.705) (-20.3276, 34.7889) (-20.3298, 35.2639) knots 0 0 0 1 1 1
  spline S1516 degree 3 poles (-20.3298, 35.2639) (-20.3899, 35.3735) (-20.4501, 35.4799) (-20.5156, 35.5873) knots 0 0 0 0 1 1 1 1
  spline S1517 degree 3 poles (-20.5156, 35.5873) (-20.5071, 35.4553) (-20.5018, 35.3231) (-20.4996, 35.1908) knots 0 0 0 0 1 1 1 1
  spline S1518 degree 2 poles (-20.4996, 35.1908) (-20.4985, 34.891) (-20.362, 34.705) knots 0 0 0 1 1 1
  spline S1519 degree 3 poles (-19.3469, 30.9107) (-19.2157, 30.7699) (-19.1052, 30.2896) (-19.0363, 29.8598) knots 0 0 0 0 1 1 1 1
  spline S1520 degree 3 poles (-19.0363, 29.8598) (-19.0299, 30.0048) (-19.0257, 30.151) (-19.0257, 30.2971) knots 0 0 0 0 1 1 1 1
  spline S1521 degree 3 poles (-19.0257, 30.2971) (-19.0257, 30.3412) (-19.0257, 30.3863) (-19.0277, 30.4293) knots 0 0 0 0 1 1 1 1
  spline S1522 degree 3 poles (-19.0277, 30.4293) (-19.0825, 30.6249) (-19.134, 30.7818) (-19.162, 30.8441) knots 0 0 0 0 1 1 1 1
  spline S1523 degree 3 poles (-19.162, 30.8441) (-19.2458, 31.0278) (-19.5488, 31.1289) (-19.3469, 30.9107) knots 0 0 0 0 1 1 1 1
  spline S1524 degree 3 poles (-25.5455, 39.1378) (-25.625, 39.832) (-25.8121, 39.9727) (-25.9259, 39.9899) knots 0 0 0 0 1 1 1 1
  spline S1525 degree 3 poles (-25.9259, 39.9899) (-25.7659, 39.6923) (-25.6745, 39.3775) (-25.653, 39.0432) knots 0 0 0 0 1 1 1 1
  spline S1526 degree 3 poles (-25.653, 39.0432) (-25.6408, 38.8722) (-25.6476, 38.7003) (-25.6734, 38.5307) knots 0 0 0 0 1 1 1 1
  spline S1527 degree 3 poles (-25.6734, 38.5307) (-25.6302, 38.2704) (-25.571, 38.0131) (-25.4962, 37.7603) knots 0 0 0 0 1 1 1 1
  spline S1528 degree 3 poles (-25.4962, 37.7603) (-25.3608, 37.7795) (-25.4275, 38.1138) (-25.5455, 39.1378) knots 0 0 0 0 1 1 1 1
  spline S1529 degree 2 poles (-22.7761, 37.8301) (-22.978, 38.2137) (-22.9275, 38.4512) knots 0 0 0 1 1 1
  spline S1530 degree 3 poles (-22.9275, 38.4512) (-22.9253, 38.4554) (-22.9253, 38.4576) (-22.9253, 38.4618) knots 0 0 0 0 1 1 1 1
  spline S1531 degree 3 poles (-22.9253, 38.4618) (-22.9586, 38.4931) (-22.9951, 38.5232) (-23.0306, 38.5543) knots 0 0 0 0 1 1 1 1
  spline S1532 degree 3 poles (-23.0306, 38.5543) (-23.0467, 38.3522) (-23.0467, 38.0676) (-22.7761, 37.8301) knots 0 0 0 0 1 1 1 1
  spline S1533 degree 3 poles (-23.9417, 22.214) (-23.9492, 21.9357) (-23.7526, 21.6241) (-23.6784, 21.5145) knots 0 0 0 0 1 1 1 1
  line L677 (-23.6784, 21.5145) -> (-23.6161, 21.5617)
  spline S1534 degree 3 poles (-23.6161, 21.5617) (-23.7, 21.6982) (-23.73, 21.9722) (-23.774, 22.1463) knots 0 0 0 0 1 1 1 1
  spline S1535 degree 3 poles (-23.774, 22.1463) (-23.8246, 22.3483) (-23.9341, 22.5579) (-23.9417, 22.214) knots 0 0 0 0 1 1 1 1
  spline S1536 degree 3 poles (-24.1264, 23.7421) (-24.1802, 23.985) (-24.3272, 23.9398) (-24.3369, 23.8119) knots 0 0 0 0 1 1 1 1
  spline S1537 degree 3 poles (-24.3369, 23.8119) (-24.2957, 23.6337) (-24.2393, 23.4594) (-24.1683, 23.2908) knots 0 0 0 0 1 1 1 1
  spline S1538 degree 3 poles (-24.1683, 23.2908) (-23.8697, 22.7062) (-23.2778, 22.1517) (-23.0909, 21.9873) knots 0 0 0 0 1 1 1 1
  line L678 (-23.0909, 21.9873) -> (-22.9489, 22.1098)
  spline S1539 degree 3 poles (-22.9489, 22.1098) (-23.7009, 22.7051) (-24.0684, 23.4734) (-24.1264, 23.7421) knots 0 0 0 0 1 1 1 1
  line L679 (-21.6587, 26.8058) -> (-21.4579, 26.6553)
  spline S1540 degree 2 poles (-21.4579, 26.6553) (-21.4664, 26.8058) (-21.6587, 26.8058) knots 0 0 0 1 1 1
  line L680 (-21.403, 26.2373) -> (-21.2022, 26.0858)
  spline S1541 degree 2 poles (-21.2022, 26.0858) (-21.2097, 26.2373) (-21.403, 26.2373) knots 0 0 0 1 1 1
  line L681 (-20.8981, 26.3351) -> (-20.7241, 26.204)
  spline S1542 degree 3 poles (-20.7241, 26.204) (-20.723, 26.204) (-20.7294, 26.3351) (-20.8981, 26.3351) knots 0 0 0 0 1 1 1 1
  line L682 (-20.8454, 25.8666) -> (-20.6435, 25.715)
  spline S1543 degree 2 poles (-20.6435, 25.715) (-20.6521, 25.8666) (-20.8454, 25.8666) knots 0 0 0 1 1 1
  line L683 (-21.2483, 26.924) -> (-21.0464, 26.7724)
  spline S1544 degree 2 poles (-21.0464, 26.7724) (-21.055, 26.924) (-21.2483, 26.924) knots 0 0 0 1 1 1
  line L684 (-21.7436, 27.343) -> (-21.5417, 27.1926)
  spline S1545 degree 2 poles (-21.5417, 27.1926) (-21.5503, 27.343) (-21.7436, 27.343) knots 0 0 0 1 1 1
  line L685 (-21.1452, 28.0802) -> (-20.9443, 27.9287)
  spline S1546 degree 2 poles (-20.9443, 27.9287) (-20.9518, 28.0802) (-21.1452, 28.0802) knots 0 0 0 1 1 1
  line L686 (-20.2514, 26.6242) -> (-20.087, 26.5017)
  spline S1547 degree 2 poles (-20.087, 26.5017) (-20.0945, 26.6242) (-20.2514, 26.6242) knots 0 0 0 1 1 1
  line L687 (-21.2505, 25.7376) -> (-21.0486, 25.5872)
  spline S1548 degree 2 poles (-21.0486, 25.5872) (-21.0572, 25.7376) (-21.2505, 25.7376) knots 0 0 0 1 1 1
  line L688 (-21.0818, 25.2938) -> (-20.8133, 25.0918)
  spline S1549 degree 2 poles (-20.8133, 25.0918) (-20.8251, 25.2938) (-21.0818, 25.2938) knots 0 0 0 1 1 1
  line L689 (-21.7242, 24.5126) -> (-21.5836, 24.4073)
  spline S1550 degree 2 poles (-21.5836, 24.4073) (-21.59, 24.5126) (-21.7242, 24.5126) knots 0 0 0 1 1 1
  line L690 (-21.8478, 25.0499) -> (-21.6469, 24.8983)
  spline S1551 degree 2 poles (-21.6469, 24.8983) (-21.6555, 25.0499) (-21.8478, 25.0499) knots 0 0 0 1 1 1
  line L691 (-20.782, 28.2898) -> (-20.5801, 28.1393)
  spline S1552 degree 3 poles (-20.5801, 28.1393) (-20.5812, 28.1393) (-20.5887, 28.2898) (-20.782, 28.2898) knots 0 0 0 0 1 1 1 1
  line L692 (-20.4469, 28.4327) -> (-20.2449, 28.2812)
  spline S1553 degree 2 poles (-20.2449, 28.2812) (-20.2535, 28.4327) (-20.4469, 28.4327) knots 0 0 0 1 1 1
  line L693 (-20.5931, 27.7063) -> (-20.4212, 27.5762)
  spline S1554 degree 2 poles (-20.4212, 27.5762) (-20.4287, 27.7063) (-20.5931, 27.7063) knots 0 0 0 1 1 1
  line L694 (-20.2911, 27.875) -> (-20.1278, 27.7525)
  spline S1555 degree 2 poles (-20.1278, 27.7525) (-20.1343, 27.875) (-20.2911, 27.875) knots 0 0 0 1 1 1
  line L695 (-19.9259, 28.0276) -> (-19.7786, 27.9169)
  spline S1556 degree 3 poles (-19.7786, 27.9169) (-19.7797, 27.9169) (-19.7852, 28.0276) (-19.9259, 28.0276) knots 0 0 0 0 1 1 1 1
  line L696 (-19.7518, 27.4935) -> (-19.6111, 27.3871)
  spline S1557 degree 2 poles (-19.6111, 27.3871) (-19.6175, 27.4935) (-19.7518, 27.4935) knots 0 0 0 1 1 1
  line L697 (-20.0559, 27.3538) -> (-19.8539, 27.2023)
  spline S1558 degree 3 poles (-19.8539, 27.2023) (-19.855, 27.2023) (-19.8636, 27.3538) (-20.0559, 27.3538) knots 0 0 0 0 1 1 1 1
  line L698 (-20.535, 27.2281) -> (-20.3331, 27.0766)
  spline S1559 degree 2 poles (-20.3331, 27.0766) (-20.3417, 27.2281) (-20.535, 27.2281) knots 0 0 0 1 1 1
  line L699 (-20.8498, 27.0508) -> (-20.694, 26.9336)
  spline S1560 degree 2 poles (-20.694, 26.9336) (-20.7005, 27.0508) (-20.8498, 27.0508) knots 0 0 0 1 1 1
  line L700 (-21.5921, 28.0168) -> (-21.3901, 27.8664)
  spline S1561 degree 2 poles (-21.3901, 27.8664) (-21.3977, 28.0168) (-21.5921, 28.0168) knots 0 0 0 1 1 1
  line L701 (-21.735, 28.5122) -> (-21.5331, 28.3618)
  spline S1562 degree 3 poles (-21.5331, 28.3618) (-21.532, 28.3618) (-21.5417, 28.5122) (-21.735, 28.5122) knots 0 0 0 0 1 1 1 1
  line L702 (-21.3407, 28.6777) -> (-21.1935, 28.567)
  spline S1563 degree 2 poles (-21.1935, 28.567) (-21.2, 28.6777) (-21.3407, 28.6777) knots 0 0 0 1 1 1
  line L703 (-21.4794, 29.2085) -> (-21.3322, 29.0979)
  spline S1564 degree 2 poles (-21.3322, 29.0979) (-21.3386, 29.2085) (-21.4794, 29.2085) knots 0 0 0 1 1 1
  line L704 (-21.6298, 29.7297) -> (-21.4825, 29.618)
  spline S1565 degree 2 poles (-21.4825, 29.618) (-21.4889, 29.7297) (-21.6298, 29.7297) knots 0 0 0 1 1 1
  line L705 (-21.8554, 30.2251) -> (-21.706, 30.1134)
  spline S1566 degree 2 poles (-21.706, 30.1134) (-21.7135, 30.2251) (-21.8554, 30.2251) knots 0 0 0 1 1 1
  line L706 (-22.8254, 31.2019) -> (-22.6783, 31.0891)
  spline S1567 degree 2 poles (-22.6783, 31.0891) (-22.6836, 31.1783) (-22.8254, 31.2019) knots 0 0 0 1 1 1
  line L707 (-23.0275, 26.3652) -> (-22.8791, 26.2523)
  spline S1568 degree 2 poles (-22.8791, 26.2523) (-22.8855, 26.3415) (-23.0275, 26.3652) knots 0 0 0 1 1 1
  line L708 (-24.0684, 25.2917) -> (-23.9202, 25.1799)
  spline S1569 degree 2 poles (-23.9202, 25.1799) (-23.9266, 25.268) (-24.0684, 25.2917) knots 0 0 0 1 1 1
  line L709 (-20.9669, 28.8357) -> (-20.7649, 28.6842)
  spline S1570 degree 2 poles (-20.7649, 28.6842) (-20.7734, 28.8357) (-20.9669, 28.8357) knots 0 0 0 1 1 1
  line L710 (-19.9677, 26.8713) -> (-19.7658, 26.7198)
  spline S1571 degree 3 poles (-19.7658, 26.7198) (-19.7669, 26.7198) (-19.7755, 26.8713) (-19.9677, 26.8713) knots 0 0 0 0 1 1 1 1
  line L711 (-20.4963, 26.0256) -> (-20.2955, 25.8741)
  spline S1572 degree 2 poles (-20.2955, 25.8741) (-20.3041, 26.0256) (-20.4963, 26.0256) knots 0 0 0 1 1 1
  line L712 (-21.663, 25.6796) -> (-21.4191, 25.4969)
  spline S1573 degree 3 poles (-21.4191, 25.4969) (-21.4202, 25.4969) (-21.4299, 25.6796) (-21.663, 25.6796) knots 0 0 0 0 1 1 1 1
  line L713 (-21.4955, 25.1519) -> (-21.2934, 25.0015)
  spline S1574 degree 3 poles (-21.2934, 25.0015) (-21.2945, 25.0015) (-21.302, 25.1519) (-21.4955, 25.1519) knots 0 0 0 0 1 1 1 1
  line L714 (-20.7069, 25.3293) -> (-20.5049, 25.1777)
  spline S1575 degree 2 poles (-20.5049, 25.1777) (-20.5135, 25.3293) (-20.7069, 25.3293) knots 0 0 0 1 1 1
  line L715 (-21.0592, 24.7834) -> (-20.8573, 24.6318)
  spline S1576 degree 3 poles (-20.8573, 24.6318) (-20.8562, 24.6318) (-20.8659, 24.7834) (-21.0592, 24.7834) knots 0 0 0 0 1 1 1 1
  line L716 (-21.4449, 24.6652) -> (-21.243, 24.5136)
  spline S1577 degree 3 poles (-21.243, 24.5136) (-21.2441, 24.5136) (-21.2527, 24.6652) (-21.4449, 24.6652) knots 0 0 0 0 1 1 1 1
  spline S1578 degree 3 poles (-39.4106, 36.9036) (-39.3268, 36.9036) (-39.243, 36.9542) (-39.1754, 36.9725) knots 0 0 0 0 1 1 1 1
  spline S1579 degree 3 poles (-39.1754, 36.9725) (-39.1087, 36.9875) (-39.0916, 37.1218) (-39.1592, 37.1068) knots 0 0 0 0 1 1 1 1
  spline S1580 degree 3 poles (-39.1592, 37.1068) (-39.2258, 37.0874) (-39.3096, 37.0563) (-39.3601, 37.0381) knots 0 0 0 0 1 1 1 1
  spline S1581 degree 3 poles (-39.3601, 37.0381) (-39.4106, 37.024) (-39.4944, 36.9036) (-39.4106, 36.9036) knots 0 0 0 0 1 1 1 1
  spline S1582 degree 3 poles (-39.5417, 36.39) (-39.4643, 36.39) (-39.3816, 36.4341) (-39.3193, 36.447) knots 0 0 0 0 1 1 1 1
  spline S1583 degree 3 poles (-39.3193, 36.447) (-39.2581, 36.4642) (-39.243, 36.5921) (-39.3053, 36.5791) knots 0 0 0 0 1 1 1 1
  spline S1584 degree 3 poles (-39.3053, 36.5791) (-39.3698, 36.5662) (-39.4482, 36.5351) (-39.4966, 36.52) knots 0 0 0 0 1 1 1 1
  spline S1585 degree 3 poles (-39.4966, 36.52) (-39.5471, 36.505) (-39.6212, 36.3879) (-39.5417, 36.39) knots 0 0 0 0 1 1 1 1
  spline S1586 degree 3 poles (-39.5879, 35.9214) (-39.517, 35.9214) (-39.4343, 35.9591) (-39.3795, 35.972) knots 0 0 0 0 1 1 1 1
  spline S1587 degree 3 poles (-39.3795, 35.972) (-39.3225, 35.987) (-39.3086, 36.1085) (-39.3687, 36.0977) knots 0 0 0 0 1 1 1 1
  spline S1588 degree 3 poles (-39.3687, 36.0977) (-39.4289, 36.0913) (-39.503, 36.0623) (-39.5481, 36.0493) knots 0 0 0 0 1 1 1 1
  spline S1589 degree 3 poles (-39.5481, 36.0493) (-39.5997, 36.0396) (-39.6631, 35.9194) (-39.5879, 35.9214) knots 0 0 0 0 1 1 1 1
  spline S1590 degree 3 poles (-40.1659, 35.7517) (-40.095, 35.7539) (-40.0466, 35.7893) (-39.9908, 35.8043) knots 0 0 0 0 1 1 1 1
  spline S1591 degree 3 poles (-39.9908, 35.8043) (-39.9349, 35.8173) (-39.9198, 35.9386) (-39.98, 35.93) knots 0 0 0 0 1 1 1 1
  spline S1592 degree 3 poles (-39.98, 35.93) (-40.0402, 35.9194) (-40.0821, 35.8946) (-40.1272, 35.8796) knots 0 0 0 0 1 1 1 1
  spline S1593 degree 3 poles (-40.1272, 35.8796) (-40.1788, 35.8699) (-40.2411, 35.7495) (-40.1659, 35.7517) knots 0 0 0 0 1 1 1 1
  spline S1594 degree 3 poles (-39.6394, 35.5153) (-39.5739, 35.5175) (-39.4923, 35.5465) (-39.4429, 35.5571) knots 0 0 0 0 1 1 1 1
  spline S1595 degree 3 poles (-39.4429, 35.5571) (-39.3924, 35.5701) (-39.3795, 35.685) (-39.4353, 35.6808) knots 0 0 0 0 1 1 1 1
  spline S1596 degree 3 poles (-39.4353, 35.6808) (-39.4923, 35.6743) (-39.5632, 35.6496) (-39.604, 35.641) knots 0 0 0 0 1 1 1 1
  spline S1597 degree 3 poles (-39.604, 35.641) (-39.6566, 35.6324) (-39.7104, 35.5109) (-39.6394, 35.5153) knots 0 0 0 0 1 1 1 1
  spline S1598 degree 3 poles (-39.6556, 35.1134) (-39.5976, 35.1177) (-39.517, 35.1402) (-39.4719, 35.1488) knots 0 0 0 0 1 1 1 1
  spline S1599 degree 3 poles (-39.4719, 35.1488) (-39.4289, 35.1596) (-39.4171, 35.2681) (-39.4697, 35.2681) knots 0 0 0 0 1 1 1 1
  spline S1600 degree 3 poles (-39.4697, 35.2681) (-39.5213, 35.2659) (-39.5879, 35.2456) (-39.6276, 35.237) knots 0 0 0 0 1 1 1 1
  spline S1601 degree 3 poles (-39.6276, 35.237) (-39.6803, 35.2316) (-39.7233, 35.1123) (-39.6556, 35.1134) knots 0 0 0 0 1 1 1 1
  spline S1602 degree 3 poles (-39.6405, 34.7319) (-39.5879, 34.7363) (-39.5084, 34.7534) (-39.4697, 34.7588) knots 0 0 0 0 1 1 1 1
  spline S1603 degree 3 poles (-39.4697, 34.7588) (-39.43, 34.7673) (-39.4203, 34.8717) (-39.4697, 34.8737) knots 0 0 0 0 1 1 1 1
  spline S1604 degree 3 poles (-39.4697, 34.8737) (-39.5181, 34.8759) (-39.5804, 34.8565) (-39.618, 34.8523) knots 0 0 0 0 1 1 1 1
  spline S1605 degree 3 poles (-39.618, 34.8523) (-39.6695, 34.8468) (-39.7028, 34.7277) (-39.6405, 34.7319) knots 0 0 0 0 1 1 1 1
  spline S1606 degree 3 poles (-39.6233, 34.3751) (-39.5771, 34.3795) (-39.4987, 34.3902) (-39.4665, 34.3945) knots 0 0 0 0 1 1 1 1
  spline S1607 degree 3 poles (-39.4665, 34.3945) (-39.4332, 34.4009) (-39.4235, 34.4977) (-39.4697, 34.5063) knots 0 0 0 0 1 1 1 1
  spline S1608 degree 3 poles (-39.4697, 34.5063) (-39.5148, 34.5127) (-39.5718, 34.4955) (-39.6051, 34.4933) knots 0 0 0 0 1 1 1 1
  spline S1609 degree 3 poles (-39.6051, 34.4933) (-39.6599, 34.4902) (-39.6824, 34.3709) (-39.6233, 34.3751) knots 0 0 0 0 1 1 1 1
  spline S1610 degree 3 poles (-39.5782, 34.0797) (-39.5385, 34.0861) (-39.4611, 34.0883) (-39.4321, 34.0925) knots 0 0 0 0 1 1 1 1
  spline S1611 degree 3 poles (-39.4321, 34.0925) (-39.4063, 34.0968) (-39.3967, 34.1871) (-39.4386, 34.2001) knots 0 0 0 0 1 1 1 1
  spline S1612 degree 3 poles (-39.4386, 34.2001) (-39.4805, 34.2107) (-39.5331, 34.1979) (-39.5642, 34.1979) knots 0 0 0 0 1 1 1 1
  spline S1613 degree 3 poles (-39.5642, 34.1979) (-39.6201, 34.1968) (-39.633, 34.0731) (-39.5782, 34.0797) knots 0 0 0 0 1 1 1 1
  spline S1614 degree 3 poles (-40.1626, 35.3841) (-40.0971, 35.3841) (-40.0509, 35.4175) (-40.0004, 35.4283) knots 0 0 0 0 1 1 1 1
  spline S1615 degree 3 poles (-40.0004, 35.4283) (-39.951, 35.4411) (-39.9381, 35.5518) (-39.9929, 35.5454) knots 0 0 0 0 1 1 1 1
  spline S1616 degree 3 poles (-39.9929, 35.5454) (-40.0477, 35.5389) (-40.0864, 35.512) (-40.1272, 35.5034) knots 0 0 0 0 1 1 1 1
  spline S1617 degree 3 poles (-40.1272, 35.5034) (-40.1766, 35.4938) (-40.2314, 35.3821) (-40.1626, 35.3841) knots 0 0 0 0 1 1 1 1
  spline S1618 degree 3 poles (-40.602, 35.9934) (-40.5365, 35.9956) (-40.4903, 36.0268) (-40.4398, 36.0396) knots 0 0 0 0 1 1 1 1
  spline S1619 degree 3 poles (-40.4398, 36.0396) (-40.3904, 36.0504) (-40.3764, 36.1611) (-40.4323, 36.1525) knots 0 0 0 0 1 1 1 1
  spline S1620 degree 3 poles (-40.4323, 36.1525) (-40.486, 36.1461) (-40.5257, 36.1235) (-40.5666, 36.1105) knots 0 0 0 0 1 1 1 1
  spline S1621 degree 3 poles (-40.5666, 36.1105) (-40.6149, 36.102) (-40.6708, 35.9914) (-40.602, 35.9934) knots 0 0 0 0 1 1 1 1
  spline S1622 degree 3 poles (-40.1358, 35.0198) (-40.0778, 35.022) (-40.0316, 35.0489) (-39.9875, 35.0575) knots 0 0 0 0 1 1 1 1
  spline S1623 degree 3 poles (-39.9875, 35.0575) (-39.9435, 35.0682) (-39.9317, 35.1693) (-39.9811, 35.1649) knots 0 0 0 0 1 1 1 1
  spline S1624 degree 3 poles (-39.9811, 35.1649) (-40.0305, 35.1607) (-40.0681, 35.1402) (-40.1046, 35.1316) knots 0 0 0 0 1 1 1 1
  spline S1625 degree 3 poles (-40.1046, 35.1316) (-40.1508, 35.1198) (-40.1981, 35.0178) (-40.1358, 35.0198) knots 0 0 0 0 1 1 1 1
  spline S1626 degree 3 poles (-40.0928, 34.6524) (-40.0434, 34.6546) (-39.9972, 34.6749) (-39.9596, 34.6835) knots 0 0 0 0 1 1 1 1
  spline S1627 degree 3 poles (-39.9596, 34.6835) (-39.9198, 34.6921) (-39.9102, 34.7825) (-39.9542, 34.7803) knots 0 0 0 0 1 1 1 1
  spline S1628 degree 3 poles (-39.9542, 34.7803) (-39.9983, 34.7781) (-40.0348, 34.7588) (-40.067, 34.7513) knots 0 0 0 0 1 1 1 1
  spline S1629 degree 3 poles (-40.067, 34.7513) (-40.11, 34.7449) (-40.1487, 34.6502) (-40.0928, 34.6524) knots 0 0 0 0 1 1 1 1
  spline S1630 degree 3 poles (-40.0563, 34.3333) (-40.0133, 34.3354) (-39.9682, 34.3526) (-39.936, 34.3579) knots 0 0 0 0 1 1 1 1
  spline S1631 degree 3 poles (-39.936, 34.3579) (-39.9037, 34.3634) (-39.8951, 34.446) (-39.9338, 34.444) knots 0 0 0 0 1 1 1 1
  spline S1632 degree 3 poles (-39.9338, 34.444) (-39.9725, 34.444) (-40.0069, 34.4288) (-40.0359, 34.4246) knots 0 0 0 0 1 1 1 1
  spline S1633 degree 3 poles (-40.0359, 34.4246) (-40.0756, 34.4191) (-40.1057, 34.3311) (-40.0563, 34.3333) knots 0 0 0 0 1 1 1 1
  spline S1634 degree 3 poles (-40.009, 33.9829) (-39.9736, 33.985) (-39.9295, 33.998) (-39.9037, 34.0022) knots 0 0 0 0 1 1 1 1
  spline S1635 degree 3 poles (-39.9037, 34.0022) (-39.8769, 34.0088) (-39.8693, 34.0775) (-39.9027, 34.0797) knots 0 0 0 0 1 1 1 1
  spline S1636 degree 3 poles (-39.9027, 34.0797) (-39.936, 34.0797) (-39.9682, 34.0689) (-39.994, 34.0645) knots 0 0 0 0 1 1 1 1
  spline S1637 degree 3 poles (-39.994, 34.0645) (-40.0294, 34.0625) (-40.0531, 33.9808) (-40.009, 33.9829) knots 0 0 0 0 1 1 1 1
  spline S1638 degree 3 poles (-41.0167, 35.4605) (-40.9802, 35.4605) (-40.9372, 35.4735) (-40.9082, 35.4777) knots 0 0 0 0 1 1 1 1
  spline S1639 degree 3 poles (-40.9082, 35.4777) (-40.8835, 35.4841) (-40.8749, 35.5529) (-40.9082, 35.5551) knots 0 0 0 0 1 1 1 1
  spline S1640 degree 3 poles (-40.9082, 35.5551) (-40.9426, 35.5571) (-40.9748, 35.5443) (-40.9995, 35.5422) knots 0 0 0 0 1 1 1 1
  spline S1641 degree 3 poles (-40.9995, 35.5422) (-41.036, 35.5378) (-41.0597, 35.4561) (-41.0167, 35.4605) knots 0 0 0 0 1 1 1 1
  spline S1642 degree 3 poles (-40.6096, 35.6302) (-40.5494, 35.6302) (-40.5032, 35.6571) (-40.457, 35.67) knots 0 0 0 0 1 1 1 1